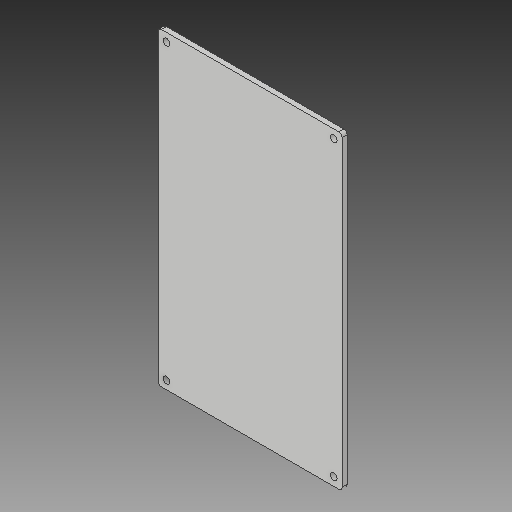
# Autodesk Inventor part: Tampa caixa principal
Saved by Autodesk Inventor 2019 (Build 230136000, 136)
## iProperties
Created: 2020-06-01
Part Number: Tampa caixa principal
Material: Generic
Document SubType Name: Modeling
Designer: luiza
Density: 1 g/cm^3
Appearance: Default
Author: luiza
Autodesk Inventor part; units mm, degrees
ref_plane "YZ Plane" through (0, 0, 0) normal (1, 0, 0) x (0, 1, 0)
ref_plane "XZ Plane" through (0, 0, 0) normal (0, 1, 0) x (-1, 0, 0)
ref_plane "XY Plane" through (0, 0, 0) normal (0, 0, 1) x (1, 0, 0)
sketch "Sketch1" plane through (0, 0, 0) normal (0, 0, 1) x (1, 0, 0)
  circle A0 centre (50, 87.5) radius 2.01 projected
  circle A1 centre (50, -87.5) radius 2.01 projected
  line L0 (55, -90.5) -> (55, 90.5) projected
  arc A2 (55, 90.5) -> (53, 92.5) centre (53, 90.5) ccw projected
  line L1 (53, 92.5) -> (-53, 92.5) projected
  arc A3 (-53, 92.5) -> (-55, 90.5) centre (-53, 90.5) ccw projected
  line L2 (-55, 90.5) -> (-55, -90.5) projected
  arc A4 (-55, -90.5) -> (-53, -92.5) centre (-53, -90.5) ccw projected
  line L3 (-53, -92.5) -> (53, -92.5) projected
  arc A5 (53, -92.5) -> (55, -90.5) centre (53, -90.5) ccw projected
  circle A6 centre (-50, 87.5) radius 2.01 projected
  circle A7 centre (-50, -87.5) radius 2.01 projected
ref_plane "Work Plane1" through (0, 0, 0) normal (0, 0, -1) x (-1, 0, 0)
sketch "Sketch2" plane through (0, 0, 0) normal (0, 0, -1) x (-1, 0, 0)
  arc A0 (-37.8653, -89.5) -> (-47, -80.3653) centre (-50, -92.5) ccw projected
  line L0 (-37.8653, -89.5) -> (37.8653, -89.5) projected
  line L1 (-47, 80.3653) -> (-47, -80.3653) projected
  arc A1 (47, -80.3653) -> (37.8653, -89.5) centre (50, -92.5) ccw projected
  line L2 (47, -80.3653) -> (47, 80.3653) projected
  arc A2 (37.8653, 89.5) -> (47, 80.3653) centre (50, 92.5) ccw projected
  line L3 (37.8653, 89.5) -> (-37.8653, 89.5) projected
  arc A3 (-47, 80.3653) -> (-37.8653, 89.5) centre (-50, 92.5) ccw projected
  line L4 (46, 79.6062) -> (46, -79.6062)
  arc A4 (46, -79.6062) -> (37.1062, -88.5) centre (50, -92.5) ccw
  line L5 (37.1062, -88.5) -> (-37.1062, -88.5)
  arc A5 (-37.1062, -88.5) -> (-46, -79.6062) centre (-50, -92.5) ccw
  line L6 (-46, -79.6062) -> (-46, 79.6062)
  arc A6 (-46, 79.6062) -> (-37.1062, 88.5) centre (-50, 92.5) ccw
  line L7 (-37.1062, 88.5) -> (37.1062, 88.5)
  arc A7 (37.1062, 88.5) -> (46, 79.6062) centre (50, 92.5) ccw
  line L8 (42, -76.9356) -> (42, 76.9356)
  arc A8 (34.4356, 84.5) -> (42, 76.9356) centre (50, 92.5) ccw
  line L9 (34.4356, 84.5) -> (-34.4356, 84.5)
  arc A9 (-42, 76.9356) -> (-34.4356, 84.5) centre (-50, 92.5) ccw
  line L10 (-42, 76.9356) -> (-42, -76.9356)
  arc A10 (-34.4356, -84.5) -> (-42, -76.9356) centre (-50, -92.5) ccw
  line L11 (-34.4356, -84.5) -> (34.4356, -84.5)
  arc A11 (42, -76.9356) -> (34.4356, -84.5) centre (50, -92.5) ccw
  dimension "d7" = 1
  dimension "d8" = 4
  constraints: 16 end point, 16 point on circle, 8 centre point, 14 other
  measures "d7" distance between parallel lines of L2 L4
  measures "d8" distance between parallel lines of L4 L8
extrude "Extrusion2" add sketch "Sketch2" along normal blind 4 contours L4 A4 L5 A5 L6 A6 L7 A7
extrude "Extrusion3" add sketch "Sketch1" along normal blind 3
body "Solid1"
